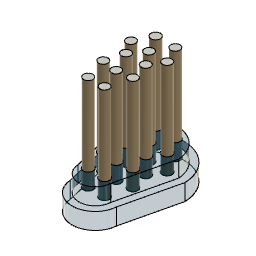
Ensamble Pie mojado (Autodesk Fusion 360 archive; units mm, degrees)
design "Molde Interior"
Autodesk Fusion 360 part; units mm, degrees
sketch "Boceto1" plane through (0, 0, 0) normal (0, 0, 1) x (1, 0, 0)
  line L0 (0, 0) -> (0, 9) construction
  arc A0 (-10, 9) -> (10, 9) centre (0, 10.0556) ccw construction
  line L1 (10, 9) -> (14, 26) construction
  arc A1 (14.9995, 25.882) -> (-14.9995, 25.882) centre (0, 26) ccw construction
  line L2 (-10, 9) -> (-14, 26) construction
  line L3 (-10, 9) -> (10, 9) construction
  line L4 (0, 40) -> (0, 26) construction
  arc A2 (-10.9875, 8.8309) -> (10.9875, 8.8309) centre (0, 10.0556) ccw construction
  line L5 (10.9875, 8.8309) -> (14.9995, 25.882) construction
  line L6 (-10.9875, 8.8309) -> (-14.9995, 25.882) construction
  arc A3 (14, 26) -> (-14, 26) centre (0, 26) ccw construction
  line L7 (-14, 26) -> (14, 26) construction
  line L8 (0, 0) -> (0, 40) construction
  arc A4 (10.9951, 26.3275) -> (-10.9951, 26.3275) centre (0, 26) ccw
  line L9 (-7.0326, 9.4867) -> (-10.9951, 26.3275)
  arc A5 (-7.0326, 9.4867) -> (7.0326, 9.4867) centre (0, 10.0556) ccw
  line L10 (7.0326, 9.4867) -> (10.9951, 26.3275)
  dimension "d1" = 1
  dimension "d2" = 40
  dimension "d3" = 9
  dimension "d4" = 14
  dimension "d5" = 28
  dimension "d6" = 20
  dimension "d7" = 3
  constraint coincident L0.start L8.start
  constraint vertical L8
  constraint parallel L0 L8
  constraint parallel L4 L8
  constraint perpendicular L4 L7
  constraint midpoint A1.centre L7
  constraint horizontal L3
  constraint midpoint L0.end L3
  constraint coincident L4.start A3
  constraint coincident L0.start A0
  measures "d2" distance of L0.start L4.start
  measures "d3" distance of L0.end L0.start
  measures "d4" distance of L4.start A1.centre
  measures "d5" distance of L1.end L2.end
  measures "d6" distance of A0.start A0.end
extrude "Extruir1" add sketch "Boceto1" along normal blind 5 makes body 1
sketch "Boceto2" plane through (0, 0, 5) normal (0, 0, 1) x (-1, 0, 0)
  arc A0 (7.0326, -9.4867) -> (-7.0326, -9.4867) centre (0, -10.0556) ccw
  line L0 (-7.0326, -9.4867) -> (-10.9951, -26.3275)
  arc A1 (-10.9951, -26.3275) -> (10.9951, -26.3275) centre (0, -26) ccw
  line L1 (10.9951, -26.3275) -> (7.0326, -9.4867)
  line L2 (8.8845, -26.5258) -> (4.949, -9.8)
  arc A2 (4.949, -9.8) -> (-4.949, -9.8) centre (0, -10.0556) ccw
  line L3 (-4.949, -9.8) -> (-8.8845, -26.5258)
  arc A3 (-8.8845, -26.5258) -> (8.8845, -26.5258) centre (0, -26) ccw
  dimension "d10" = -2.1
extrude "Extruir2" add sketch "Boceto2" along normal blind 5 contours L2 A2 L3 A3 bodies 1
sketch "Boceto3" plane through (0, 0, 10) normal (0, 0, 1) x (-1, 0, 0)
  arc A0 (-8.8845, -26.5258) -> (8.8845, -26.5258) centre (0, -26) ccw
  line L0 (8.8845, -26.5258) -> (4.949, -9.8)
  arc A1 (4.949, -9.8) -> (-4.949, -9.8) centre (0, -10.0556) ccw
  line L1 (-4.949, -9.8) -> (-8.8845, -26.5258)
  line L2 (0, -34.9) -> (0, -5.1) construction
  line L3 (0, -20) -> (7.349, -20) construction
  line L4 (0, -20) -> (-7.349, -20) construction
  circle A2 centre (3, -31.4) radius 1.5
  line L5 (0, -34.9) -> (0, -31.4) construction
  line L6 (0, -31.4) -> (3, -31.4) construction
  circle A3 centre (-3, -31.4) radius 1.5
  line L7 (0, -34.9) -> (0, -26.4) construction
  line L8 (0, -26.4) -> (5.5, -26.4) construction
  circle A4 centre (5.5, -26.4) radius 1.5
  circle A5 centre (-5.5, -26.4) radius 1.5
  circle A6 centre (0, -26.4) radius 1.5
  circle A7 centre (3, -22.4) radius 1.5
  circle A8 centre (-3, -22.4) radius 1.5
  circle A9 centre (0, -16.4) radius 1.5
  circle A10 centre (-3, -10.4) radius 1.5 construction
  circle A11 centre (3, -10.4) radius 1.5 construction
  circle A12 centre (5.5, -17) radius 1.5 construction
  circle A13 centre (-5.5, -17) radius 1.5 construction
  line L9 (5.5, -17) -> (4.5, -17) construction
  circle A14 centre (4.5, -17) radius 1.5
  line L10 (-5.5, -17) -> (-4.5, -17) construction
  circle A15 centre (-4.5, -17) radius 1.5
  line L11 (3, -10.4) -> (2.5, -10.4) construction
  line L12 (-3, -10.4) -> (-2.5, -10.4) construction
  circle A16 centre (2.5, -10.4) radius 1.5
  circle A17 centre (-2.5, -10.4) radius 1.5
  dimension "d13" = 3
  dimension "d14" = 3.5
  dimension "d15" = 3
  dimension "d16" = 3
  dimension "d17" = 3
  dimension "d18" = 5
  dimension "d21" = 0
  dimension "d22" = 9
  dimension "d25" = 0
  dimension "d26" = 10
  dimension "d29" = 0
  dimension "d30" = 21
  dimension "d35" = 5.5
  dimension "d38" = 1
  dimension "d39" = 3
  dimension "d40" = 3
  dimension "d41" = 0.5
  dimension "d42" = 0.5
  dimension "d43" = 3
  dimension "d44" = 3
  dimension "d45" = 1
  constraint midpoint A0 L2.start
  constraint midpoint A1 L2.end
  constraint midpoint L2 L3.start
  constraint coincident L0 L3.end
  constraint perpendicular L2 L3
  constraint coincident L1 L4.end
  constraint perpendicular L2 L4
  constraint parallel L2 L5
  constraint perpendicular L5 L6
  constraint symmetric L2 A2 A3
  constraint coincident L2 L7.end
  constraint parallel L2 L7
  constraint perpendicular L7 L8
  constraint coincident L8.end A4.centre
  constraint symmetric L2 A4 A5
  constraint coincident L7.end L8.start
  constraint coincident A2.centre L6.end
  constraint coincident A12.centre L9.start
  constraint perpendicular L2 L9
  constraint coincident L9.end A14.centre
  constraint coincident A13.centre L10.start
  constraint horizontal L10
  constraint coincident L10.end A15.centre
  constraint coincident A11.centre L11.start
  constraint perpendicular L2 L11
  constraint coincident A10.centre L12.start
  constraint horizontal L12
  constraint coincident L11.end A16.centre
  constraint coincident L12.end A17.centre
  measures "d13" diameter of A2
  measures "d14" distance of L2.start L5.end
  measures "d15" distance of L5.end A2.centre
  measures "d16" diameter of A4
  measures "d17" diameter of A6
  measures "d18" distance of L5.end L7.end
  measures "d35" distance of L7.end L8.end
  measures "d38" distance of A12.centre L9.end
  measures "d39" diameter of A14
  measures "d40" diameter of A15
  measures "d41" distance of A10.centre L12.end
  measures "d42" distance of A11.centre L11.end
  measures "d43" diameter of A16
  measures "d44" diameter of A17
  measures "d45" distance of A13.centre L10.end
extrude "Extruir3" add sketch "Boceto3" along normal blind 24 separate body contours A2 | A3 | A4 | A5 | A6 | A7 | A8 | A9 | A14 | A15 | A16 | A17 makes body 2 at (3.0019, 17.0748, 26) makes body 3 at (4.0019, 26.4748, 26) makes body 4 at (1.5019, 22.4748, 26) makes body 5 at (-4.4981, 22.4748, 26) makes body 6 at (4.4095, 31.913, 26) makes body 7 at (-3.9981, 10.4748, 26) makes body 8 at (-5.9981, 17.0748, 26) makes body 9 at (-6.9981, 26.4748, 26) makes body 10 at (-1.4981, 16.4748, 26) makes body 11 at (-1.4981, 26.4748, 26) makes body 12 at (-1.5905, 31.913, 26) makes body 13 at (1.0019, 10.4748, 26)
extrude "Extruir4" cut sketch "Boceto3" against normal blind 5 contours A2 | A3 | A4 | A5 | A6 | A7 | A8 | A9 | A14 | A15 | A16 | A17 bodies 1
extrude "Extruir5" add 12 faces at (-2.084, 10.2947, 10) (-2.75, 23.2669, 10) (-4.2334, 15.9775, 10) (-0.4671, 16.6898, 10) (2.6931, 10.7148, 10) (4.0495, 16.9321, 10) (3.25, 23.2669, 10) (0.25, 27.2669, 10) (-5.9944, 27.1547, 10) (-2.7722, 31.9804, 10) (3.1605, 32.0128, 10) (5.0329, 26.6898, 10) along direction (0, 0, -1) blind 5 on bodies 2 3 4 5 6 7 8 9 10 11 12 13 bodies 7 2 3 4 5 6 8 9 10 11 12 13
sketch "Boceto4" plane through (0, 0, 34) normal (0, 0, 1) x (-1, 0, 0)
  circle A0 centre (2.5, -10.4) radius 1.5
  circle A1 centre (-2.5, -10.4) radius 1.5
  circle A2 centre (0, -16.4) radius 1.5
  circle A3 centre (4.5, -17) radius 1.5
  circle A4 centre (-4.5, -17) radius 1.5
  circle A5 centre (-3, -22.4) radius 1.5
  circle A6 centre (3, -22.4) radius 1.5
  circle A7 centre (0, -26.4) radius 1.5
  circle A8 centre (-5.5, -26.4) radius 1.5
  circle A9 centre (-3, -31.4) radius 1.5
  circle A10 centre (3, -31.4) radius 1.5
  circle A11 centre (5.5, -26.4) radius 1.5
  circle A12 centre (4.5, -17) radius 1.5
  circle A13 centre (3, -31.4) radius 1.45
  circle A14 centre (-3, -31.4) radius 1.4
  circle A15 centre (5.5, -26.4) radius 1.4
  circle A16 centre (0, -26.4) radius 1.4
  circle A17 centre (-5.5, -26.4) radius 1.4
  circle A18 centre (3, -22.4) radius 1.4
  circle A19 centre (-3, -22.4) radius 1.4
  circle A20 centre (4.5, -17) radius 1.4
  circle A21 centre (0, -16.4) radius 1.4
  circle A22 centre (-4.5, -17) radius 1.4
  circle A23 centre (2.5, -10.4) radius 1.4
  circle A24 centre (-2.5, -10.4) radius 1.4
  dimension "d50" = 2.9
  dimension "d51" = -0.1
  dimension "d52" = -0.1
  dimension "d53" = -0.1
  dimension "d54" = -0.1
  dimension "d55" = -0.1
  dimension "d56" = -0.1
  dimension "d57" = -0.1
  dimension "d58" = -0.1
  dimension "d59" = -0.1
  dimension "d60" = -0.1
  dimension "d61" = -0.1
  constraint concentric A10 A13
  measures "d50" diameter of A13
extrude "Extruir6" cut sketch "Boceto4" against normal blind 29.5 bodies 2 3 4 5 6 7 8 9 10 11 12 13

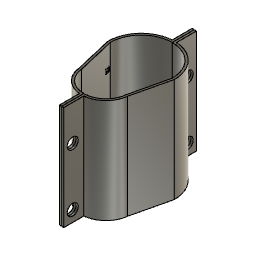
design "Molde Exterior"
Autodesk Fusion 360 part; units mm, degrees
sketch "Boceto1" plane through (0, 0, 0) normal (0, 0, 1) x (1, 0, 0)
  line L0 (0, 0) -> (0, 40)
  line L1 (0, 0) -> (0, 9) construction
  line L2 (0, 40) -> (0, 26) construction
  line L3 (-14, 26) -> (14, 26) construction
  line L4 (-10, 9) -> (10, 9) construction
  arc A0 (14, 26) -> (-14, 26) centre (0, 26) ccw
  arc A1 (-10, 9) -> (10, 9) centre (0, 10.055556) ccw
  line L5 (-10, 9) -> (-14, 26)
  line L6 (10, 9) -> (14, 26)
  line L7 (-10.987514, 8.830871) -> (-14.999536, 25.881964)
  arc A2 (14.999536, 25.881964) -> (-14.999536, 25.881964) centre (0, 26) ccw
  line L8 (10.987514, 8.830871) -> (14.999536, 25.881964)
  arc A3 (-10.987514, 8.830871) -> (10.987514, 8.830871) centre (0, 10.055556) ccw
  line L9 (-7.032583, 9.486666) -> (-10.995125, 26.327467) construction
  arc A4 (10.995125, 26.327467) -> (-10.995125, 26.327467) centre (0, 26) ccw
  line L10 (7.032583, 9.486666) -> (10.995125, 26.327467) construction
  arc A5 (-7.032583, 9.486666) -> (7.032583, 9.486666) centre (0, 10.055556) ccw
  line L11 (-0.5, 37.500001) -> (0.5, 37.500001)
  line L12 (-0.5, 37.500001) -> (-0.5, 36.98863)
  line L13 (0.5, 37.500001) -> (0.5, 36.98863)
  line L14 (0.5, 2.75) -> (-0.5, 2.75)
  line L15 (-0.5, 2.75) -> (-0.5, 3.017739)
  line L16 (0.5, 3.017739) -> (0.5, 2.75)
  line L17 (0.5, 2.75) -> (0, 3) construction
  line L18 (-0.5, 2.75) -> (0, 3) construction
  dimension "d1" = 40
  dimension "d2" = 9
  dimension "d3" = 14
  dimension "d4" = 28
  dimension "d5" = 20
  dimension "d6" = 1
  dimension "d38" = -3
  constraint coincident L0.start L1.start
  constraint vertical L0
  constraint parallel L0 L1
  constraint parallel L0 L2
  constraint perpendicular L2 L3
  constraint midpoint L2.end L3
  constraint horizontal L4
  constraint midpoint L1.end L4
  constraint coincident L0.end A0
  constraint coincident L0.start A1
  constraint horizontal L11
  constraint perpendicular L11 L12
  constraint perpendicular L11 L13
  constraint horizontal L14
  constraint perpendicular L14 L15
  constraint parallel L15 L16
  constraint midpoint A5 L17.end
  measures "d1" distance of L0.start L0.end
  measures "d2" distance of L0.start L1.end
  measures "d3" distance of L0.end L2.end
  measures "d4" distance of L3.start L3.end
  measures "d5" distance of L4.start L4.end
extrude "Extruir1" add sketch "Boceto1" against normal blind 1 contours L0 A0 A1 L5 A4 A5 L11 L12 L14 L15 | L0 A0 A1 L6 A4 A5 L11 L13 L14 L16 | L0 A5 L14 L15 | L0 A5 L14 L16 | L0 A4 L11 L12 | L0 A4 L11 L13 | L7 A2 L8 A3 picked at (-3.333333, 16.333333) picked at (3.333333, 16.333333) picked at (-0.222264, 2.833991) picked at (0.222264, 2.833991) picked at (-0.222239, 37.332913) picked at (0.222239, 37.332913) picked at (-13.329016, 20.237611) makes body 1
extrude "Extruir2" add sketch "Boceto1" along normal blind 35 contours L7 A2 L8 A3 picked at (-13.329016, 20.237611) bodies 1
ref_plane "PlanoDeObra1" through (0, 18.864476, 17) normal (1, 0, 0) x (0, -1, 0)
split "Dividir1" by plane through (0, 18.864476, 17) normal (1, 0, 0) bodies 1 makes body 2 at (10.392529, 36.816438, 11)
sketch "Boceto2" plane through (0, 0, 0) normal (1, 0, 0) x (0, 1, 0)
  line L0 (-1, 35) -> (-1, -1)
  line L1 (-1, -1) -> (-10, -1)
  line L2 (-10, -1) -> (-10, 35)
  line L3 (-10, 35) -> (-1, 35)
  line L4 (41, -1) -> (41, 35)
  line L5 (41, -1) -> (50, -1)
  line L6 (50, -1) -> (50, 35)
  line L7 (50, 35) -> (41, 35)
  dimension "d11" = 9
  dimension "d12" = 9
  constraint coincident L0.end L1.start
  constraint perpendicular L0 L1
  constraint perpendicular L1 L2
  constraint coincident L0.start L3.end
  constraint perpendicular L0 L3
  constraint coincident L4.start L5.start
  constraint perpendicular L4 L5
  constraint perpendicular L5 L6
  constraint coincident L4.end L7.end
  constraint perpendicular L4 L7
  measures "d11" distance of L0.end L1.end
  measures "d12" distance of L4.start L5.end
extrude "Extruir3" add sketch "Boceto2" along normal blind 1 separate body contours L0 L1 L2 L3 | L4 L5 L6 L7 picked at (-7, 23) picked at (44, 11) makes body 3 at (0, 44, 11) makes body 4 at (0, -7, 23)
extrude "Extruir4" add 1 faces at (0.333333, -1, 23) along direction (0, 1, 0) blind 0.24 on bodies 4 bodies 2 3 4
extrude "Extruir5" add 1 faces at (0.333333, 41, 11) along direction (0, -1, 0) blind 0.2 on bodies 3 bodies 2 3
extrude "Extruir6" add sketch "Boceto2" against normal blind 1 contours L0 L1 L2 L3 | L4 L5 L6 L7 picked at (-7, 23) picked at (44, 11) bodies 1
extrude "Extruir7" add 1 faces at (-0.333333, -1, 23) along direction (0, 1, 0) blind 0.2 on bodies 1 bodies 1
extrude "Extruir8" add 1 faces at (-0.666667, 41, 23) along direction (0, -1, 0) blind 0.2 on bodies 1 bodies 1
sketch "Boceto3" plane through (-1, 0, 0) normal (-1, 0, 0) x (0, -1, 0)
  line L0 (-50, -1) -> (-40.96663, -1)
  line L1 (-40.96663, -1) -> (-40.96663, 35)
  line L2 (-40.96663, 35) -> (-50, 35)
  line L3 (-50, 35) -> (-50, -1)
  line L4 (-50, -1) -> (-50, 35)
  line L5 (10, -1) -> (10, 35)
  line L6 (-50, -1) -> (-46, -1)
  line L7 (-46, -1) -> (-46, 4) construction
  line L8 (-50, 35) -> (-46, 35) construction
  line L9 (-46, 35) -> (-46, 30) construction
  circle A0 centre (-46, 30) radius 2.5
  circle A1 centre (-46, 4) radius 2.5
  line L10 (10, 35) -> (6, 35)
  line L11 (6, 35) -> (6, 30) construction
  line L12 (10, -1) -> (6, -1) construction
  line L13 (6, -1) -> (6, 4) construction
  circle A2 centre (6, 30) radius 2.5
  circle A3 centre (6, 4) radius 2.5
  dimension "d25" = 4
  dimension "d26" = 5
  dimension "d27" = 4
  dimension "d28" = 5
  dimension "d29" = 5
  dimension "d30" = 5
  dimension "d31" = 4
  dimension "d32" = 5
  dimension "d33" = 5
  dimension "d34" = 5
  dimension "d35" = 5
  constraint coincident L0.start L3.end
  constraint perpendicular L4 L6
  constraint perpendicular L6 L7
  constraint coincident L2.end L3.start
  constraint perpendicular L4 L8
  constraint perpendicular L8 L9
  constraint coincident L9.end A0.centre
  constraint coincident L7.end A1.centre
  constraint coincident L5.end L10.start
  constraint perpendicular L5 L10
  constraint perpendicular L10 L11
  constraint coincident L5.start L12.start
  constraint perpendicular L5 L12
  constraint perpendicular L12 L13
  constraint coincident L11.end A2.centre
  constraint coincident L13.end A3.centre
  measures "d25" distance of L0.start L6.end
  measures "d26" distance of L6.end L7.end
  measures "d27" distance of L2.end L8.end
  measures "d28" distance of L8.end L9.end
  measures "d29" diameter of A0
  measures "d30" diameter of A1
  measures "d31" distance of L5.end L10.end
  measures "d32" distance of L10.end L11.end
  measures "d33" distance of L12.end L13.end
  measures "d34" diameter of A2
  measures "d35" diameter of A3
extrude "Extruir9" cut sketch "Boceto3" against normal blind 2 contours A0 | A1 | A2 | A3 picked at (-45.265964, 30.585374) picked at (-46.366726, 4.055275) picked at (6.627353, 28.633411) picked at (5.893318, 4.289956) bodies 1 2
extrude "Extruir10" add sketch "Boceto1" along normal blind 1 contours L0 A5 L14 L15 | L0 A4 L11 L12 picked at (-0.222264, 2.833991) picked at (-0.222239, 37.332913) bodies 1
extrude "Extruir11" add sketch "Boceto1" along normal blind 1 contours L0 A5 L14 L16 | L0 A4 L11 L13 picked at (0.222264, 2.833991) picked at (0.222239, 37.332913) bodies 2
ref_plane "PlanoDeObra2" through (-7.555411, 20, 35) normal (0, 0, 1) x (1, 0, 0)
extrude "Extruir12" add 1 faces at (-0.333333, 43.655543, 35) along direction (0, 0, 1) blind 11 on bodies 1 bodies 1
extrude "Extruir13" add 1 faces at (0.333333, 43.655543, 35) along direction (0, 0, 1) blind 11 on bodies 2 bodies 2
sketch "Boceto4" plane through (0, 0, 35) normal (0, 0, 1) x (1, 0, 0)
  line L0 (0, 40) -> (0, 50)
  line L1 (0, 50) -> (-1, 50)
  line L2 (-1, 50) -> (-1, 40.96663)
  arc A0 (-1, 40.96663) -> (-14.999536, 25.881964) centre (0, 26) ccw
  line L3 (-14.999536, 25.881964) -> (-10.987514, 8.830871)
  arc A1 (-10.987514, 8.830871) -> (-1, -0.954681) centre (0, 10.055556) ccw
  line L4 (-1, -0.954681) -> (-1, -10)
  line L5 (-1, -10) -> (0, -10)
  line L6 (0, -10) -> (0, 0)
  arc A2 (-10, 9) -> (0, 0) centre (0, 10.055556) ccw
  line L7 (-10, 9) -> (-14, 26)
  arc A3 (0, 40) -> (-14, 26) centre (0, 26) ccw
  line L8 (-13.392959, 23.420074) -> (-11.446124, 23.878153)
  line L9 (-11.446124, 23.878153) -> (-11.904203, 25.824987)
  line L10 (-11.904203, 25.824987) -> (-13.851037, 25.366909)
  dimension "d51" = 2
  dimension "d52" = 2
  constraint perpendicular L7 L8
  constraint perpendicular L8 L9
  constraint perpendicular L7 L10
extrude "Extruir14" add sketch "Boceto4" along normal blind 2 contours L7 L8 L9 L10 picked at (-13.0494, 24.870657) bodies 1
extrude "Extruir15" cut 1 faces at (-11.598817, 24.527098, 35.666667) along direction (-0.97341717, -0.22903933, 0) blind 2.5 on bodies 1 bodies 1
